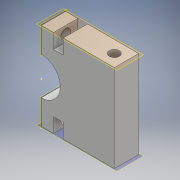
# Autodesk Inventor part: BIKE
Saved by Autodesk Inventor 2018 (Build 220112000, 112)
## iProperties
Created: 2017-05-26
Part Number: BIKE
Material: Generic
Document SubType Name: Modeling
Designer: Zadeka
Density: 1 g/cm^3
Appearance: Default
Author: Zadeka
Autodesk Inventor part; units mm, degrees
ref_plane "YZ Plane" through (0, 0, 0) normal (1, 0, 0) x (0, 1, 0)
ref_plane "XZ Plane" through (0, 0, 0) normal (0, 1, 0) x (-1, 0, 0)
ref_plane "XY Plane" through (0, 0, 0) normal (0, 0, 1) x (1, 0, 0)
sketch "Sketch1" plane through (0, 0, 0) normal (0, 1, 0) x (-1, 0, 0)
  circle A0 centre (2.1306, 2.1694) radius 15.5
  line L0 (2.1306, 17.6694) -> (2.1306, 38.1694)
  line L1 (2.1306, -13.3306) -> (2.1306, -33.8306)
  line L2 (2.1306, 38.1694) -> (-57.8694, 38.1694)
  line L3 (2.1306, -33.8306) -> (-57.8694, -33.8306)
  line L4 (-57.8694, -33.8306) -> (-57.8694, 38.1694)
  line L5 (2.1306, 38.1694) -> (34.8074, 38.1694)
  line L6 (34.8074, 38.1694) -> (34.8074, -33.8306)
  line L7 (34.8074, -33.8306) -> (2.1306, -33.8306)
  circle A1 centre (2.1306, 2.1694) radius 15.25
  point P0 (0, 0)
  dimension "d0" = 31
  dimension "d1" = 20.5
  dimension "d2" = 20.5
  dimension "d3" = 60
  dimension "d4" = 30.5
  constraints: 16 end point, 4 perpendicular, 2 centre point, 2 horizontal, 2 point on circle, 2 vertical, 1 coincident
  measures "d0" diameter of A0
  measures "d1" distance of L0.start L0.end
  measures "d2" distance of L1.start L1.end
  measures "d3" distance of L0.end L2.end
  measures "d4" diameter of A1
extrude "Extrusion1" add sketch "Sketch1" along normal blind 20 contours A0 L1 L3 L4 L2 L0
ref_plane "Work Plane1" through (-2.1306, 0, 38.1694) normal (0, 0, 1) x (1, 0, 0)
sketch "Sketch2" plane through (-2.1306, 0, 38.1694) normal (0, 0, 1) x (1, 0, 0)
  line L0 (60, 0) -> (60, 20) projected
  line L1 (60, 10) -> (50, 10)
  circle A0 centre (50, 10) radius 4.1
  point P0 (2.1306, 0)
  dimension "d31" = 8.2
  constraints: 2 end point, 1 centre point, 1 coincident, 1 horizontal, 1 midpoint
  measures "d31" diameter of A0
extrude "Extrusion2" cut sketch "Sketch2" against normal blind 192.5
ref_plane "Work Plane2" through (-2.1306, 0, 17.6694) normal (-1, 0, 0) x (0, 0, 1)
sketch "Sketch3" plane through (-2.1306, 0, 17.6694) normal (-1, 0, 0) x (0, 0, 1)
  point P0 (-17.6694, 0)
sketch "Sketch4" plane through (-2.1306, 0, 17.6694) normal (-1, 0, 0) x (0, 0, 1)
  line L0 (20.5, 0) -> (20.5, 20) projected
  circle A0 centre (14.5, 10) radius 4
  point P0 (-17.6694, 0)
  dimension "d14" = 8
  constraints: 1 centre point
  measures "d14" diameter of A0
sketch "Sketch5" plane through (-2.1306, 0, 38.1694) normal (0, 0, 1) x (1, 0, 0)
  line L0 (0, 0) -> (0, 20) projected
  line L1 (60, 0) -> (0, 0) projected
  line L2 (10, 0) -> (18, 0)
  line L3 (18, 0) -> (18, 20.6661)
  line L4 (18, 20.6661) -> (10, 20.6661)
  line L5 (10, 20.6661) -> (10, 0)
  point P0 (2.1306, 0)
  dimension "d16" = 8
  constraints: 8 end point, 2 parallel, 1 horizontal, 1 perpendicular, 1 point on line
  measures "d16" distance of L4.end L3.end
extrude "Extrusion3" cut sketch "Sketch5" against normal blind 12
extrude "Extrusion4" cut sketch "Sketch4" against normal blind 12.5
ref_plane "Work Plane3" through (-2.1306, 0, -33.8306) normal (-1, 0, 0) x (0, 0, 1)
sketch "Sketch6" plane through (-2.1306, 0, -33.8306) normal (-1, 0, 0) x (0, 0, 1)
  line L0 (0, 6) -> (0, 14) projected
  circle A0 centre (6, 10) radius 4
  point P0 (33.8306, 0)
  dimension "d23" = 8
  constraints: 1 centre point
  measures "d23" diameter of A0
ref_plane "Work Plane4" through (57.8694, 0, -33.8306) normal (0, 0, -1) x (-1, 0, 0)
sketch "Sketch7" plane through (57.8694, 0, -33.8306) normal (0, 0, -1) x (-1, 0, 0)
  line L0 (60, 0) -> (60, 20) projected
  line L1 (50, 0) -> (50, 20) projected
  line L2 (50, 10) -> (50, 20)
  line L3 (0, 0) -> (60, 0) projected
  line L4 (50, 20) -> (42, 20)
  line L5 (42, 20) -> (42, 0)
  line L6 (42, 0) -> (50, 0)
  line L7 (50, 0) -> (50, 20)
  point P0 (57.8694, 0)
  dimension "d26" = 8
  constraints: 10 end point, 2 parallel, 1 horizontal, 1 perpendicular, 1 point on line
  measures "d26" distance of L6.end L5.end
extrude "Extrusion5" cut sketch "Sketch7" against normal blind 12
extrude "Extrusion6" cut sketch "Sketch6" against normal blind 11.75
body "Solid1"
